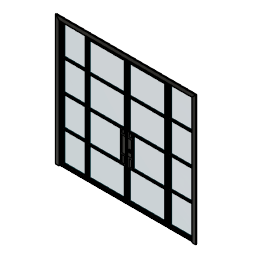
WineDoorModel (Autodesk Fusion 360 design; units mm, degrees)
Autodesk Fusion 360 part; units mm, degrees
note: some values were not read from the file. Set by a fixed rule: which sketch regions a step uses.
(part 1 of 2)
sketch "SubFloor+Framing" plane through (0, 0, 0) normal (0, 1, 0) x (1, 0, 0)
  line L0 (-1333.5, 0) -> (1333.5, 0)
  line L1 (1333.5, 0) -> (1333.5, -2514.6)
  line L2 (-1333.5, 0) -> (-1333.5, -2514.6)
  line L3 (-1333.5, -2514.6) -> (1333.5, -2514.6)
  dimension "d3" = 2667
  dimension "d4" = 2514.6
  dimension "d5" = 2514.6
  constraint horizontal L0
  constraint midpoint origin L0
  constraint perpendicular L0 L1
  constraint perpendicular L0 L2
  measures "d3" distance of L0.start L0.end
  measures "d4" distance of L0.end L1.end
  measures "d5" distance of L0.start L2.end
sketch "FinalOpening" plane through (0, 0, 0) normal (0, 1, 0) x (1, 0, 0)
  line L0 (-1333.5, 0) -> (-1333.5, -2514.6)
  line L1 (-1333.5, -2514.6) -> (1333.5, -2514.6)
  line L2 (1333.5, 0) -> (1333.5, -2514.6)
  line L3 (-1319.2125, 0) -> (-1319.2125, -2500.3125)
  line L4 (-1319.2125, -2500.3125) -> (1319.2125, -2500.3125)
  line L5 (1319.2125, 0) -> (1319.2125, -2500.3125)
  line L6 (-1333.5, 0) -> (1333.5, 0)
  line L7 (-1333.5, -19.05) -> (1333.5, -19.05)
  dimension "d9" = 19.05
sketch "Framing" plane through (0, 0, 0) normal (0, 1, 0) x (1, 0, 0)
  line L0 (-1319.2125, -2500.3125) -> (1319.2125, -2500.3125)
  line L1 (-1319.2125, 0) -> (-1319.2125, -2500.3125)
  line L2 (1319.2125, 0) -> (1319.2125, -2500.3125)
  line L3 (1293.8125, 0) -> (1293.8125, -2474.9125)
  line L4 (-1293.8125, -2474.9125) -> (1293.8125, -2474.9125)
  line L5 (-1293.8125, 0) -> (-1293.8125, -2474.9125)
  line L6 (-1370.0125, 0) -> (-1370.0125, -2551.1125)
  line L7 (-1370.0125, -2551.1125) -> (1370.0125, -2551.1125)
  line L8 (1370.0125, 0) -> (1370.0125, -2551.1125)
  line L9 (-1370.0125, 0) -> (-1293.8125, 0)
  line L10 (1293.8125, 0) -> (1370.0125, 0)
  line L11 (1293.8125, -2474.9125) -> (1370.0125, -2551.1125)
  line L12 (-1370.0125, -2551.1125) -> (-1293.8125, -2474.9125)
  line L13 (1293.8125, -19.05) -> (1370.0125, -19.05)
  line L14 (-1333.5, -19.05) -> (1333.5, -19.05)
  line L15 (-1293.8125, -19.05) -> (-1370.0125, -19.05)
  dimension "d11" = 25.4
  dimension "d12" = 50.8
  constraint perpendicular L6 L9
  constraint perpendicular L8 L10
  constraint coincident L3 L13.start
  constraint coincident L8 L13.end
  constraint perpendicular L8 L13
  constraint collinear L13 L14
  constraint coincident L5 L15.start
  constraint coincident L14 L15.start
  constraint coincident L6 L15.end
  constraint perpendicular L6 L15
sketch "1/2 Bar" plane through (0, 0, 0) normal (0, 1, 0) x (1, 0, 0)
  line L0 (-1293.8125, 0) -> (-1293.8125, -2474.9125)
  line L1 (-1293.8125, -2474.9125) -> (1293.8125, -2474.9125)
  line L2 (1293.8125, 0) -> (1293.8125, -2474.9125)
  line L3 (-1333.5, -19.05) -> (1333.5, -19.05)
  line L4 (-1281.1125, 0) -> (-1281.1125, -2462.2125)
  line L5 (-1281.1125, -2462.2125) -> (1281.1125, -2462.2125)
  line L6 (1281.1125, 0) -> (1281.1125, -2462.2125)
  line L7 (-1333.5, -31.75) -> (1333.5, -31.75)
  line L8 (-1319.2125, -2500.3125) -> (1319.2125, -2500.3125)
  line L9 (-1281.1125, -31.75) -> (-1281.1125, -2462.2125)
  line L10 (0, -2462.2125) -> (0, -31.75)
  line L11 (-787.4, -2462.2125) -> (-787.4, -31.75)
  line L12 (-800.1, -2462.2125) -> (-800.1, -31.75)
  line L13 (787.4, -2462.2125) -> (787.4, -31.75)
  line L14 (800.1, -2462.2125) -> (800.1, -31.75)
  dimension "d13" = -12.7
  dimension "d14" = 12.7
  dimension "d50" = 787.4
  dimension "d51" = 12.7
  dimension "d52" = 787.4
  dimension "d53" = 12.7
  constraint coincident L7 L9.start
  constraint coincident L4 L9.start
  constraint midpoint L5 L10.start
  constraint midpoint L7 L10.end
  constraint perpendicular L7 L10
  constraint coincident L5 L11.start
  constraint coincident L7 L11.end
  constraint perpendicular L7 L11
  constraint coincident L5 L12.start
  constraint coincident L7 L12.end
  constraint perpendicular L7 L12
  constraint coincident L5 L13.start
  constraint coincident L7 L13.end
  constraint perpendicular L7 L13
  constraint coincident L5 L14.start
  constraint coincident L7 L14.end
  constraint perpendicular L7 L14
  measures "d50" distance of L10 L11
  measures "d51" distance of L11 L12
  measures "d52" distance of L10 L13
  measures "d53" distance of L13 L14
sketch "SideLights" plane through (0, 0, 0) normal (0, 1, 0) x (1, 0, 0)
  line L0 (-1281.1125, -31.75) -> (-800.1, -31.75)
  line L1 (-800.1, -31.75) -> (-800.1, -2462.2125)
  line L2 (-800.1, -2462.2125) -> (-1281.1125, -2462.2125)
  line L3 (-1281.1125, -2462.2125) -> (-1281.1125, -31.75)
  line L4 (-1249.3625, -63.5) -> (-831.85, -63.5)
  line L5 (-831.85, -2430.4625) -> (-1249.3625, -2430.4625)
  line L6 (-1249.3625, -2430.4625) -> (-1249.3625, -1862.5344)
  line L7 (-1249.3625, -1231.1063) -> (-831.85, -1231.1063)
  line L8 (-1249.3625, -1262.8563) -> (-831.85, -1262.8563)
  line L9 (-1249.3625, -1830.7844) -> (-831.85, -1830.7844)
  line L10 (-1249.3625, -1862.5344) -> (-831.85, -1862.5344)
  line L11 (-1249.3625, -631.4281) -> (-1249.3625, -63.5)
  line L12 (-1249.3625, -1231.1063) -> (-1249.3625, -663.1781)
  line L13 (-1249.3625, -1830.7844) -> (-1249.3625, -1262.8563)
  line L14 (-831.85, -63.5) -> (-831.85, -631.4281)
  line L15 (-831.85, -663.1781) -> (-831.85, -1231.1063)
  line L16 (-831.85, -1262.8563) -> (-831.85, -1830.7844)
  line L17 (-831.85, -1862.5344) -> (-831.85, -2430.4625)
  line L18 (-1249.3625, -663.1781) -> (-831.85, -663.1781)
  line L19 (-1249.3625, -631.4281) -> (-831.85, -631.4281)
  line L20 (0, -2462.2125) -> (0, -31.75)
  line L21 (1249.3625, -1862.5344) -> (831.85, -1862.5344)
  line L22 (831.85, -1862.5344) -> (831.85, -2430.4625)
  line L23 (1249.3625, -2430.4625) -> (1249.3625, -1862.5344)
  line L24 (831.85, -2430.4625) -> (1249.3625, -2430.4625)
  line L25 (800.1, -31.75) -> (800.1, -2462.2125)
  line L26 (800.1, -2462.2125) -> (1281.1125, -2462.2125)
  line L27 (1249.3625, -1830.7844) -> (831.85, -1830.7844)
  line L28 (1281.1125, -31.75) -> (800.1, -31.75)
  line L29 (1249.3625, -663.1781) -> (831.85, -663.1781)
  line L30 (1249.3625, -1231.1062) -> (831.85, -1231.1062)
  line L31 (1249.3625, -1830.7844) -> (1249.3625, -1262.8562)
  line L32 (831.85, -1262.8562) -> (831.85, -1830.7844)
  line L33 (1249.3625, -631.4281) -> (831.85, -631.4281)
  line L34 (1249.3625, -63.5) -> (831.85, -63.5)
  line L35 (1281.1125, -2462.2125) -> (1281.1125, -31.75)
  line L36 (1249.3625, -631.4281) -> (1249.3625, -63.5)
  line L37 (831.85, -63.5) -> (831.85, -631.4281)
  line L38 (1249.3625, -1262.8562) -> (831.85, -1262.8562)
  line L39 (831.85, -663.1781) -> (831.85, -1231.1062)
  line L40 (1249.3625, -1231.1062) -> (1249.3625, -663.1781)
  line L41 (-1040.6062, -2430.4625) -> (-1040.6062, -2462.2125)
  point P0 (-1281.1125, -31.75)
  point P1 (-800.1, -31.75)
  point P2 (-800.1, -2462.2125)
  point P3 (-1281.1125, -2462.2125)
  point P4 (800.1, -2462.2125)
  point P5 (800.1, -31.75)
  point P6 (1281.1125, -2462.2125)
  point P7 (1281.1125, -31.75)
  dimension "d56" = 31.75
  dimension "d57" = 31.75
  dimension "d58" = 31.75
  dimension "d124" = 31.75
  dimension "d129" = 567.9281
  dimension "d130" = 567.9281
  dimension "d131" = 567.9281
  dimension "d132" = 567.9281
  constraint coincident P0 L0.start
  constraint coincident P1 L0.end
  constraint coincident P2 L1.end
  constraint coincident P3 L2.end
  constraint coincident L15.start L14
  constraint coincident L7.end L14
  constraint perpendicular L7 L14
  constraint coincident L8.end L14
  constraint perpendicular L8 L14
  constraint coincident L9.end L14
  constraint perpendicular L9 L14
  constraint coincident L10.end L14
  constraint perpendicular L10 L14
  constraint coincident L12.end L11
  constraint coincident L8.start L12
  constraint coincident L6.end L13
  constraint collinear L14 L15
  constraint collinear L15 L16
  constraint collinear L16 L17
  constraint collinear L6 L13
  constraint perpendicular L15 L18
  constraint perpendicular L14 L19
  constraint collinear L11 L12
  constraint symmetric P0 L20 P7
  constraint symmetric P1 L20 P5
  constraint symmetric P2 L20 P4
  constraint symmetric P3 L20 P6
  constraint symmetric L4.start L20 L34.start
  constraint symmetric L4.end L20 L34.end
  constraint symmetric L5.start L20 L22.end
  constraint symmetric L5.end L20 L23.start
  constraint symmetric L11.start L20 L33.start
  constraint symmetric L14.end L20 L33.end
  constraint symmetric L12.end L20 L29.start
  constraint symmetric L15.start L20 L29.end
  constraint symmetric L7.start L20 L30.start
  constraint symmetric L7.end L20 L30.end
  constraint symmetric L8.start L20 L31.end
  constraint symmetric L8.end L20 L32.start
  constraint symmetric L9.start L20 L27.start
  constraint symmetric L9.end L20 L27.end
  constraint symmetric L6.end L20 L21.start
  constraint symmetric L10.end L20 L21.end
  constraint midpoint L5 L41.start
  constraint midpoint L2 L41.end
  constraint perpendicular L4 L11
  measures "d56" distance of L7 L8
  measures "d57" distance of L9 L10
  measures "d58" distance of L18 L19
  measures "d124" distance of L41.start L41.end
  measures "d129" distance of L5 L10
  measures "d130" distance of L4.start L11.start
  measures "d131" distance of L12.end L7.start
  measures "d132" distance of L8.start L9.start
sketch "Doors" plane through (0, 0, 0) normal (0, 1, 0) x (1, 0, 0)
  line L0 (-787.4, -31.75) -> (787.4, -31.75)
  line L1 (787.4, -31.75) -> (787.4, -2462.2125)
  line L2 (787.4, -2462.2125) -> (-787.4, -2462.2125)
  line L3 (-787.4, -2462.2125) -> (-787.4, -31.75)
  line L4 (-787.4, -2462.2125) -> (-787.4, -31.75)
  line L5 (782.6375, -41.275) -> (782.6375, -2457.45)
  line L6 (782.6375, -2457.45) -> (-782.6375, -2457.45)
  line L7 (-782.6375, -2457.45) -> (-782.6375, -41.275)
  line L8 (-3.175, -41.275) -> (3.175, -41.275)
  line L9 (0, -2457.45) -> (0, -41.275)
  line L10 (3.175, -2457.45) -> (3.175, -41.275)
  line L11 (-3.175, -2457.45) -> (-3.175, -41.275)
  line L12 (3.175, -41.275) -> (782.6375, -41.275)
  line L13 (-782.6375, -41.275) -> (-3.175, -41.275)
  line L14 (-15.875, -2444.75) -> (-769.9375, -2444.75)
  line L15 (-769.9375, -2444.75) -> (-769.9375, -53.975)
  line L16 (-769.9375, -53.975) -> (-15.875, -53.975)
  line L17 (-15.875, -2444.75) -> (-15.875, -53.975)
  line L18 (-738.1875, -85.725) -> (-47.625, -85.725)
  line L19 (-47.625, -2413) -> (-738.1875, -2413)
  line L20 (-738.1875, -631.4281) -> (-47.625, -631.4281)
  line L21 (-738.1875, -1262.8563) -> (-47.625, -1262.8562)
  line L22 (-738.1875, -1830.7844) -> (-47.625, -1830.7844)
  line L23 (-738.1875, -1862.5344) -> (-47.625, -1862.5344)
  line L24 (-1249.3625, -631.4281) -> (-831.85, -631.4281)
  line L25 (-1249.3625, -663.1781) -> (-831.85, -663.1781)
  line L26 (-1249.3625, -1231.1063) -> (-831.85, -1231.1063)
  line L27 (-1249.3625, -1262.8563) -> (-831.85, -1262.8563)
  line L28 (-1249.3625, -1830.7844) -> (-831.85, -1830.7844)
  line L29 (-1249.3625, -1862.5344) -> (-831.85, -1862.5344)
  line L30 (-738.1875, -631.4281) -> (-738.1875, -85.725)
  line L31 (-47.625, -631.4281) -> (-47.625, -85.725)
  line L32 (-738.1875, -1231.1063) -> (-738.1875, -663.1781)
  line L33 (-47.625, -2413) -> (-47.625, -1862.5344)
  line L34 (-47.625, -1830.7844) -> (-47.625, -1262.8562)
  line L35 (-738.1875, -2413) -> (-738.1875, -1862.5344)
  line L36 (-738.1875, -1830.7844) -> (-738.1875, -1262.8563)
  line L37 (15.875, -2444.75) -> (15.875, -53.975)
  line L38 (738.1875, -85.725) -> (47.625, -85.725)
  line L39 (47.625, -631.4281) -> (47.625, -85.725)
  line L40 (769.9375, -53.975) -> (15.875, -53.975)
  line L41 (738.1875, -1262.8563) -> (47.625, -1262.8562)
  line L42 (738.1875, -1231.1063) -> (738.1875, -663.1781)
  line L43 (738.1875, -1830.7844) -> (738.1875, -1262.8563)
  line L44 (47.625, -1830.7844) -> (47.625, -1262.8562)
  line L45 (738.1875, -631.4281) -> (47.625, -631.4281)
  line L46 (738.1875, -631.4281) -> (738.1875, -85.725)
  line L47 (769.9375, -2444.75) -> (769.9375, -53.975)
  line L48 (15.875, -2444.75) -> (769.9375, -2444.75)
  line L49 (738.1875, -2413) -> (738.1875, -1862.5344)
  line L50 (47.625, -2413) -> (738.1875, -2413)
  line L51 (47.625, -2413) -> (47.625, -1862.5344)
  line L52 (738.1875, -1830.7844) -> (47.625, -1830.7844)
  line L53 (738.1875, -1862.5344) -> (47.625, -1862.5344)
  line L54 (125.4125, -1231.1062) -> (125.4125, -663.1781)
  line L55 (47.625, -1167.6063) -> (93.6625, -1167.6063)
  line L56 (93.6625, -1167.6063) -> (93.6625, -1231.1062)
  line L57 (15.875, -1135.8563) -> (93.6625, -1135.8563)
  line L58 (47.625, -1231.1062) -> (47.625, -1167.6063)
  line L59 (47.625, -663.1781) -> (47.625, -799.3063)
  line L60 (15.875, -831.0563) -> (93.6625, -831.0563)
  line L61 (47.625, -799.3063) -> (93.6625, -799.3063)
  line L62 (93.6625, -1135.8563) -> (93.6625, -831.0563)
  line L63 (93.6625, -799.3063) -> (93.6625, -663.1781)
  line L64 (738.1875, -663.1781) -> (125.4125, -663.1781)
  line L65 (93.6625, -663.1781) -> (47.625, -663.1781)
  line L66 (738.1875, -1231.1063) -> (125.4125, -1231.1062)
  line L67 (93.6625, -1231.1062) -> (47.625, -1231.1062)
  line L68 (-47.625, -663.1781) -> (-47.625, -799.3063)
  line L69 (-93.6625, -663.1781) -> (-47.625, -663.1781)
  line L70 (-93.6625, -799.3063) -> (-93.6625, -663.1781)
  line L71 (-47.625, -799.3063) -> (-93.6625, -799.3063)
  line L72 (-93.6625, -1167.6063) -> (-93.6625, -1231.1062)
  line L73 (-93.6625, -1231.1062) -> (-47.625, -1231.1062)
  line L74 (-47.625, -1167.6063) -> (-93.6625, -1167.6063)
  line L75 (-47.625, -1231.1062) -> (-47.625, -1167.6063)
  line L76 (-93.6625, -1135.8563) -> (-93.6625, -831.0563)
  line L77 (-15.875, -1135.8563) -> (-93.6625, -1135.8563)
  line L78 (-15.875, -831.0563) -> (-93.6625, -831.0563)
  line L79 (-125.4125, -1231.1062) -> (-125.4125, -663.1781)
  line L80 (-47.625, -799.3063) -> (-47.625, -663.1781)
  line L81 (-738.1875, -663.1781) -> (-125.4125, -663.1781)
  line L82 (-93.6625, -663.1781) -> (-47.625, -663.1781)
  line L83 (-47.625, -1231.1062) -> (-47.625, -1167.6063)
  line L84 (-738.1875, -1231.1063) -> (-125.4125, -1231.1062)
  line L85 (-93.6625, -1231.1062) -> (-47.625, -1231.1062)
  point P0 (-787.4, -31.75)
  point P1 (787.4, -31.75)
  point P2 (787.4, -2462.2125)
  point P3 (-787.4, -2462.2125)
  dimension "d100" = 3.175
  dimension "d111" = 109.5375
  dimension "d113" = 31.75
  dimension "d114" = 63.5
  dimension "d115" = 31.75
  dimension "d116" = 31.75
  dimension "d117" = 304.8
  constraint coincident P0 L0.start
  constraint coincident P1 L0.end
  constraint coincident P2 L1.end
  constraint coincident P3 L2.end
  constraint midpoint L6 L9.start
  constraint coincident L6 L10.start
  constraint coincident L6 L11.start
  constraint coincident L8 L9.end
  constraint coincident L8.start L12
  constraint coincident L9.end L13
  constraint vertical L9
  constraint coincident L20.start L35
  constraint coincident L20.end L33
  constraint perpendicular L20 L33
  constraint perpendicular L33 L81
  constraint coincident L32.start L35
  constraint coincident L73.end L33
  constraint perpendicular L33 L84
  constraint perpendicular L21 L33
  constraint coincident L22.start L35
  constraint coincident L22.end L33
  constraint perpendicular L22 L33
  constraint perpendicular L23 L33
  constraint collinear L20 L24
  constraint collinear L25 L81
  constraint collinear L26 L84
  constraint collinear L21 L27
  constraint collinear L22 L28
  constraint collinear L23 L29
  constraint collinear L30 L35
  constraint collinear L31 L33
  constraint collinear L32 L35
  constraint collinear L33 L83
  constraint collinear L33 L34
  constraint collinear L35 L36
  constraint symmetric L9 L14.start L37.start
  constraint symmetric L9 L14.end L47.start
  constraint symmetric L9 L15.end L40.start
  constraint symmetric L9 L16.end L37.end
  constraint symmetric L9 L18.start L38.start
  constraint symmetric L9 L18.end L38.end
  constraint symmetric L9 L19.start L50.start
  constraint symmetric L9 L19.end L49.start
  constraint symmetric L9 L20.start L45.start
  constraint symmetric L9 L20.end L39.start
  constraint symmetric L9 L32.end L42.end
  constraint symmetric L9 L68.start L59.start
  constraint symmetric L9 L32.start L42.start
  constraint symmetric L9 L73.end L58.start
  constraint symmetric L9 L21.start L41.start
  constraint symmetric L9 L21.end L41.end
  constraint symmetric L9 L22.start L43.start
  constraint symmetric L9 L22.end L44.start
  constraint symmetric L9 L23.start L49.end
  constraint symmetric L9 L23.end L51.end
  constraint perpendicular L54 L64
  constraint perpendicular L54 L55
  constraint coincident L56.end L66
  constraint perpendicular L56 L66
  constraint coincident L37 L57.start
  constraint perpendicular L54 L57
  constraint perpendicular L55 L58
  constraint perpendicular L57 L62
  constraint collinear L56 L62
  constraint perpendicular L59 L64
  constraint coincident L63.end L64
  constraint coincident L37 L60.start
  constraint perpendicular L54 L60
  constraint coincident L61.end L62
  constraint perpendicular L61 L62
  constraint collinear L62 L63
  constraint collinear L64 L65
  constraint collinear L66 L67
  constraint symmetric L9 L59.start L68.start
  constraint symmetric L9 L58.start L73.end
  constraint symmetric L9 L55.end L72.start
  constraint symmetric L9 L56.end L72.end
  constraint symmetric L9 L57.start L77.start
  constraint symmetric L9 L55.start L74.start
  constraint symmetric L9 L57.end L76.start
  constraint symmetric L9 L63.end L69.start
  constraint symmetric L9 L60.start L78.start
  constraint symmetric L9 L59.end L68.end
  constraint symmetric L9 L61.end L70.start
  constraint symmetric L9 L60.end L76.end
  constraint symmetric L9 L54.start L79.start
  constraint symmetric L9 L54.end L79.end
  constraint collinear L80 L83
  constraint collinear L81 L82
  constraint collinear L84 L85
  measures "d100" distance of L9 L10
  measures "d111" distance of L37 L54
  measures "d113" distance of L54 L56
  measures "d114" distance of L55 L66
  measures "d115" distance of L55 L57
  measures "d116" distance of L60 L61
  measures "d117" distance of L57 L60
extrude "Extrude1" add sketch "Framing" against normal blind 19.05 contours L1 L6 L12 L14 L15 | L1 L5 L12 L14 L15 | L2 L3 L11 L13 L14 | L2 L8 L11 L13 L14 makes body 1 at (-1344.6125, 0, 1681.6917) makes body 2 at (1344.6125, 0, 1681.6917)
extrude "Extrude2" add sketch "Framing" against normal blind 19.05 separate body contours L0 L4 L11 L12 | L0 L7 L11 L12 makes body 3
extrude "Extrude3" add sketch "1/2 Bar" along normal blind 76.2 separate body contours L0 L3 L4 L7 | L0 L1 L2 L4 L5 L6 L7 L9 | L3 L4 L6 L7 | L2 L3 L6 L7 makes body 4
extrude "Extrude4" add sketch "1/2 Bar" along normal blind 76.2 separate body contours L5 L7 L11 L12 | L5 L7 L13 L14 makes body 5 at (-787.4, 50.8, 1652.0583) makes body 6 at (800.1, 50.8, 1652.0583)
extrude "Extrude6" add sketch "SideLights" along normal blind 4.7625 from surface at 26.9875 separate body makes body 7 at (1270.5292, 26.9875, 1041.7969) makes body 8 at (-1270.5292, 26.9875, 1041.7969)
extrude "Extrude7" add sketch "Doors" along normal blind 38.1 separate body contours L5 L6 L10 L12 | L6 L7 L11 L13 makes body 9 at (-3.175, 12.7, 1652.0583) makes body 10 at (782.6375, 12.7, 846.6667)
extrude "Extrude8" add sketch "Doors" along normal blind 4.7625 from surface at 7.9375 separate body contours L14 L15 L16 L17 L76 L77 L78 | L37 L40 L47 L48 L57 L60 L62 makes body 11 at (759.3542, 7.9375, 1453.7531) makes body 12 at (-759.3542, 7.9375, 1453.7531)
sketch "Door Handle Plates" plane through (0, 7.9375, 0) normal (0, -1, 0) x (1, 0, 0)
  line L0 (15.875, 2444.75) -> (15.875, 1135.8563)
  line L1 (15.875, 1254.9187) -> (117.475, 1254.9187)
  line L2 (15.875, 831.0563) -> (15.875, 53.975)
  line L3 (15.875, 639.3656) -> (117.475, 639.3656)
  line L4 (117.475, 1254.9187) -> (117.475, 639.3656)
  line L5 (47.625, 1262.8562) -> (738.1875, 1262.8563)
  line L6 (738.1875, 631.4281) -> (47.625, 631.4281)
  line L7 (15.875, 1254.9187) -> (15.875, 639.3656)
  line L8 (0, 2457.45) -> (0, 41.275)
  line L9 (-15.875, 639.3656) -> (-117.475, 639.3656)
  line L10 (-15.875, 1254.9187) -> (-15.875, 639.3656)
  line L11 (-15.875, 1254.9187) -> (-117.475, 1254.9187)
  line L12 (-117.475, 1254.9187) -> (-117.475, 639.3656)
  point P0 (-15.875, 1135.8563)
  point P1 (-47.625, 1262.8562)
  point P2 (-47.625, 631.4281)
  point P3 (-15.875, 831.0563)
  dimension "d118" = 101.6
  dimension "d119" = 101.6
  dimension "d120" = 7.9375
  dimension "d121" = 7.9375
  constraint coincident L0 L1.start
  constraint perpendicular L0 L1
  constraint horizontal L3
  constraint coincident L2 L3.start
  constraint perpendicular L3 L4
  constraint symmetric L0.end L8 P0
  constraint symmetric L1.start L8 L10.start
  constraint symmetric L1.end L8 L11.end
  constraint symmetric L2.start L8 P3
  constraint symmetric L3.start L8 L9.start
  constraint symmetric L3.end L8 L9.end
  constraint symmetric L5.start L8 P1
  constraint symmetric L6.end L8 P2
  measures "d118" distance of L3.start L3.end
  measures "d119" distance of L1.start L1.end
  measures "d120" distance of L1 L5
  measures "d121" distance of L3 L6
extrude "Extrude9" add sketch "Door Handle Plates" along normal blind 4.7625 separate body makes body 13 at (49.7417, 7.9375, 1049.7344) makes body 14 at (-49.7417, 7.9375, 844.55)
copy_body "CopyPasteBodies1" bodies 12 8 11 7 makes body 15 makes body 16 makes body 17 makes body 18
move_body "Move1" bodies 15 16 17 18 to x (1, 0, 0) y (0, 1, 0) z (0, 0, 1) at (0, 17.4625, 0)
sketch "Sidelight Glass" plane through (0, 31.75, 0) normal (0, 1, 0) x (-1, 0, 0)
  line L0 (-831.85, 63.5) -> (-1249.3625, 63.5)
  line L1 (-831.85, 631.4281) -> (-831.85, 63.5)
  line L2 (-1249.3625, 631.4281) -> (-831.85, 631.4281)
  line L3 (-1249.3625, 63.5) -> (-1249.3625, 631.4281)
  line L4 (-831.85, 663.1781) -> (-1249.3625, 663.1781)
  line L5 (-831.85, 1231.1062) -> (-831.85, 663.1781)
  line L6 (-1249.3625, 1231.1062) -> (-831.85, 1231.1062)
  line L7 (-1249.3625, 663.1781) -> (-1249.3625, 1231.1062)
  line L8 (-831.85, 1262.8562) -> (-1249.3625, 1262.8562)
  line L9 (-831.85, 1830.7844) -> (-831.85, 1262.8562)
  line L10 (-1249.3625, 1830.7844) -> (-831.85, 1830.7844)
  line L11 (-1249.3625, 1262.8562) -> (-1249.3625, 1830.7844)
  line L12 (-1249.3625, 1862.5344) -> (-1249.3625, 2430.4625)
  line L13 (-831.85, 1862.5344) -> (-1249.3625, 1862.5344)
  line L14 (-831.85, 2430.4625) -> (-831.85, 1862.5344)
  line L15 (-1249.3625, 2430.4625) -> (-831.85, 2430.4625)
  line L16 (-800.1, 2462.2125) -> (-1281.1125, 2462.2125)
  line L17 (-800.1, 31.75) -> (-800.1, 2462.2125)
  line L18 (-1281.1125, 31.75) -> (-800.1, 31.75)
  line L19 (-1281.1125, 2462.2125) -> (-1281.1125, 31.75)
  line L20 (-815.975, 2438.4) -> (-815.975, 1854.5969)
  line L21 (-1265.2375, 2438.4) -> (-815.975, 2438.4)
  line L22 (-1265.2375, 1854.5969) -> (-1265.2375, 2438.4)
  line L23 (-815.975, 1854.5969) -> (-1265.2375, 1854.5969)
  line L24 (-815.975, 1838.7219) -> (-815.975, 1254.9187)
  line L25 (-1265.2375, 1254.9187) -> (-1265.2375, 1838.7219)
  line L26 (-815.975, 1239.0437) -> (-815.975, 655.2406)
  line L27 (-1265.2375, 655.2406) -> (-1265.2375, 1239.0437)
  line L28 (-1265.2375, 55.5625) -> (-1265.2375, 639.3656)
  line L29 (-815.975, 639.3656) -> (-815.975, 55.5625)
  line L30 (-1265.2375, 639.3656) -> (-815.975, 639.3656)
  line L31 (-815.975, 55.5625) -> (-1265.2375, 55.5625)
  line L32 (-815.975, 655.2406) -> (-1265.2375, 655.2406)
  line L33 (-1265.2375, 1239.0437) -> (-815.975, 1239.0437)
  line L34 (-815.975, 1254.9187) -> (-1265.2375, 1254.9187)
  line L35 (-1265.2375, 1838.7219) -> (-815.975, 1838.7219)
  line L36 (0, 2457.45) -> (0, 41.275)
  line L37 (1265.2375, 655.2406) -> (1265.2375, 1239.0437)
  line L38 (815.975, 1239.0437) -> (815.975, 655.2406)
  line L39 (1281.1125, 31.75) -> (800.1, 31.75)
  line L40 (1265.2375, 1239.0437) -> (815.975, 1239.0437)
  line L41 (1265.2375, 1254.9187) -> (1265.2375, 1838.7219)
  line L42 (831.85, 1231.1063) -> (831.85, 663.1781)
  line L43 (1249.3625, 1262.8562) -> (1249.3625, 1830.7844)
  line L44 (1265.2375, 55.5625) -> (1265.2375, 639.3656)
  line L45 (1281.1125, 2462.2125) -> (1281.1125, 31.75)
  line L46 (800.1, 31.75) -> (800.1, 2462.2125)
  line L47 (831.85, 1262.8563) -> (1249.3625, 1262.8562)
  line L48 (815.975, 655.2406) -> (1265.2375, 655.2406)
  line L49 (1249.3625, 63.5) -> (1249.3625, 631.4281)
  line L50 (831.85, 631.4281) -> (831.85, 63.5)
  line L51 (1249.3625, 1231.1062) -> (831.85, 1231.1063)
  line L52 (815.975, 1254.9188) -> (1265.2375, 1254.9187)
  line L53 (815.975, 55.5625) -> (1265.2375, 55.5625)
  line L54 (800.1, 2462.2125) -> (1281.1125, 2462.2125)
  line L55 (815.975, 1854.5969) -> (1265.2375, 1854.5969)
  line L56 (815.975, 1838.7219) -> (815.975, 1254.9188)
  line L57 (815.975, 639.3656) -> (815.975, 55.5625)
  line L58 (1249.3625, 631.4281) -> (831.85, 631.4281)
  line L59 (1265.2375, 1854.5969) -> (1265.2375, 2438.4)
  line L60 (831.85, 1830.7844) -> (831.85, 1262.8563)
  line L61 (815.975, 2438.4) -> (815.975, 1854.5969)
  line L62 (1265.2375, 1838.7219) -> (815.975, 1838.7219)
  line L63 (1249.3625, 1862.5344) -> (1249.3625, 2430.4625)
  line L64 (1249.3625, 663.1781) -> (1249.3625, 1231.1062)
  line L65 (1249.3625, 1830.7844) -> (831.85, 1830.7844)
  line L66 (1249.3625, 2430.4625) -> (831.85, 2430.4625)
  line L67 (831.85, 1862.5344) -> (1249.3625, 1862.5344)
  line L68 (831.85, 2430.4625) -> (831.85, 1862.5344)
  line L69 (831.85, 663.1781) -> (1249.3625, 663.1781)
  line L70 (1265.2375, 2438.4) -> (815.975, 2438.4)
  line L71 (1265.2375, 639.3656) -> (815.975, 639.3656)
  line L72 (831.85, 63.5) -> (1249.3625, 63.5)
  line L73 (-800.1, 31.75) -> (-800.1, 2462.2125)
  dimension "d183" = 15.875
  dimension "d184" = 15.875
  dimension "d185" = 15.875
  dimension "d186" = 15.875
  dimension "d187" = 15.875
  dimension "d188" = 15.875
  dimension "d189" = 15.875
  dimension "d190" = 15.875
  dimension "d200" = 23.8125
  dimension "d201" = 23.8125
  dimension "d203" = 15.875
  dimension "d204" = 7.9375
  dimension "d205" = 7.9375
  dimension "d206" = 7.9375
  dimension "d207" = 7.9375
  dimension "d208" = 7.9375
  constraint symmetric L0.start L36 L50.end
  constraint symmetric L0.end L36 L49.start
  constraint symmetric L1.start L36 L50.start
  constraint symmetric L2.start L36 L49.end
  constraint symmetric L4.start L36 L42.end
  constraint symmetric L4.end L36 L64.start
  constraint symmetric L5.start L36 L42.start
  constraint symmetric L6.start L36 L51.start
  constraint symmetric L8.start L36 L47.start
  constraint symmetric L8.end L36 L43.start
  constraint symmetric L9.start L36 L60.start
  constraint symmetric L10.start L36 L43.end
  constraint symmetric L12.start L36 L63.start
  constraint symmetric L12.end L36 L63.end
  constraint symmetric L13.start L36 L67.start
  constraint symmetric L14.start L36 L66.end
  constraint symmetric L16.start L36 L46.end
  constraint symmetric L16.end L36 L45.start
  constraint symmetric L17.start L36 L39.end
  constraint symmetric L18.start L36 L39.start
  constraint symmetric L20.start L36 L61.start
  constraint symmetric L21.start L36 L59.end
  constraint symmetric L22.start L36 L55.end
  constraint symmetric L20.end L36 L55.start
  constraint symmetric L24.start L36 L56.start
  constraint symmetric L25.end L36 L41.end
  constraint symmetric L25.start L36 L41.start
  constraint symmetric L24.end L36 L52.start
  constraint symmetric L26.start L36 L38.start
  constraint symmetric L27.end L36 L37.end
  constraint symmetric L27.start L36 L37.start
  constraint symmetric L26.end L36 L38.end
  constraint symmetric L29.start L36 L57.start
  constraint symmetric L28.end L36 L44.end
  constraint symmetric L28.start L36 L44.start
  constraint symmetric L29.end L36 L53.start
  measures "d183" distance of L19 L22
  measures "d184" distance of L19 L25
  measures "d185" distance of L19 L27
  measures "d186" distance of L19 L28
  measures "d187" distance of L17 L29
  measures "d188" distance of L17 L26
  measures "d189" distance of L24 L73
  measures "d190" distance of L20 L73
  measures "d200" distance of L16 L21
  measures "d201" distance of L18 L31
  measures "d203" distance of L33 L34
  measures "d204" distance of L8 L34
  measures "d205" distance of L2 L30
  measures "d206" distance of L4 L32
  measures "d207" distance of L10 L35
  measures "d208" distance of L13 L23
extrude "Extrude10" add sketch "Sidelight Glass" along normal blind 6.35 separate body contours L0 L1 L2 L3 | L4 L5 L6 L7 | L8 L9 L10 L11 | L12 L13 L14 L15 | L20 L21 L22 L23 | L24 L25 L34 L35 | L26 L27 L32 L33 | L28 L29 L30 L31 | L37 L38 L40 L48 | L41 L52 L56 L62 | L42 L51 L64 L69 | L43 L47 L60 L65 | L44 L53 L57 L71 | L49 L50 L58 L72 | L55 L59 L61 L70 | L63 L66 L67 L68 makes body 19 at (-965.7292, 31.75, 1644.1208) makes body 20 at (965.7292, 31.75, 1044.4427) makes body 21 at (965.7292, 31.75, 1644.1208) makes body 22 at (-965.7292, 31.75, 1044.4427) makes body 23 at (-965.7292, 31.75, 2243.799) makes body 24 at (965.7292, 31.75, 444.7646) makes body 25 at (965.7292, 31.75, 2243.799) makes body 26 at (-965.7292, 31.75, 444.7646)
sketch "DoorGlass" plane through (0, 12.7, 0) normal (0, 1, 0) x (-1, 0, 0)
  line L0 (-47.625, 1167.6063) -> (-93.6625, 1167.6063)
  line L1 (-47.625, 1231.1062) -> (-47.625, 1167.6063)
  line L2 (-93.6625, 1231.1062) -> (-47.625, 1231.1062)
  line L3 (-93.6625, 1167.6063) -> (-93.6625, 1231.1062)
  line L4 (-125.4125, 1231.1062) -> (-125.4125, 663.1781)
  line L5 (-738.1875, 1231.1063) -> (-125.4125, 1231.1062)
  line L6 (-738.1875, 663.1781) -> (-738.1875, 1231.1063)
  line L7 (-125.4125, 663.1781) -> (-738.1875, 663.1781)
  line L8 (-47.625, 799.3063) -> (-47.625, 663.1781)
  line L9 (-93.6625, 799.3063) -> (-47.625, 799.3063)
  line L10 (-93.6625, 663.1781) -> (-93.6625, 799.3063)
  line L11 (-738.1875, 1862.5344) -> (-738.1875, 2413)
  line L12 (-47.625, 1862.5344) -> (-738.1875, 1862.5344)
  line L13 (-47.625, 2413) -> (-47.625, 1862.5344)
  line L14 (-738.1875, 2413) -> (-47.625, 2413)
  line L15 (-47.625, 1830.7844) -> (-47.625, 1262.8562)
  line L16 (-738.1875, 1830.7844) -> (-47.625, 1830.7844)
  line L17 (-738.1875, 1262.8563) -> (-738.1875, 1830.7844)
  line L18 (-47.625, 1262.8562) -> (-738.1875, 1262.8563)
  line L19 (-738.1875, 85.725) -> (-738.1875, 631.4281)
  line L20 (-47.625, 85.725) -> (-738.1875, 85.725)
  line L21 (-47.625, 631.4281) -> (-47.625, 85.725)
  line L22 (-738.1875, 631.4281) -> (-47.625, 631.4281)
  line L23 (-15.875, 2444.75) -> (-15.875, 1135.8563)
  line L24 (-15.875, 1135.8563) -> (-93.6625, 1135.8563)
  line L25 (-93.6625, 1135.8563) -> (-93.6625, 831.0563)
  line L26 (-15.875, 831.0563) -> (-93.6625, 831.0563)
  line L27 (-15.875, 831.0563) -> (-15.875, 53.975)
  line L28 (-769.9375, 53.975) -> (-15.875, 53.975)
  line L29 (-769.9375, 2444.75) -> (-769.9375, 53.975)
  line L30 (-15.875, 2444.75) -> (-769.9375, 2444.75)
  line L31 (125.4125, 1231.1062) -> (738.1875, 1231.1063)
  line L32 (125.4125, 663.1781) -> (125.4125, 1231.1062)
  line L33 (738.1875, 663.1781) -> (125.4125, 663.1781)
  line L34 (738.1875, 1231.1063) -> (738.1875, 663.1781)
  line L35 (47.625, 1167.6063) -> (47.625, 1231.1062)
  line L36 (93.6625, 1167.6063) -> (47.625, 1167.6063)
  line L37 (93.6625, 1231.1062) -> (93.6625, 1167.6063)
  line L38 (47.625, 1231.1062) -> (93.6625, 1231.1062)
  line L39 (93.6625, 799.3063) -> (93.6625, 663.1781)
  line L40 (47.625, 799.3063) -> (93.6625, 799.3063)
  line L41 (47.625, 663.1781) -> (47.625, 799.3063)
  line L42 (738.1875, 1262.8563) -> (47.625, 1262.8562)
  line L43 (738.1875, 1830.7844) -> (738.1875, 1262.8563)
  line L44 (47.625, 1830.7844) -> (738.1875, 1830.7844)
  line L45 (47.625, 1262.8562) -> (47.625, 1830.7844)
  line L46 (738.1875, 1862.5344) -> (47.625, 1862.5344)
  line L47 (738.1875, 2413) -> (738.1875, 1862.5344)
  line L48 (47.625, 2413) -> (738.1875, 2413)
  line L49 (47.625, 1862.5344) -> (47.625, 2413)
  line L50 (47.625, 85.725) -> (47.625, 631.4281)
  line L51 (738.1875, 85.725) -> (47.625, 85.725)
  line L52 (738.1875, 631.4281) -> (738.1875, 85.725)
  line L53 (47.625, 631.4281) -> (738.1875, 631.4281)
  line L54 (15.875, 2444.75) -> (769.9375, 2444.75)
  line L55 (769.9375, 2444.75) -> (769.9375, 53.975)
  line L56 (769.9375, 53.975) -> (15.875, 53.975)
  line L57 (15.875, 831.0563) -> (15.875, 53.975)
  line L58 (15.875, 831.0563) -> (93.6625, 831.0563)
  line L59 (93.6625, 1135.8563) -> (93.6625, 831.0563)
  line L60 (15.875, 1135.8563) -> (93.6625, 1135.8563)
  line L61 (15.875, 2444.75) -> (15.875, 1135.8563)
  line L62 (-31.75, 1838.7219) -> (-31.75, 1254.9187)
  line L63 (-31.75, 2420.9375) -> (-31.75, 1854.5969)
  line L64 (-754.0625, 1854.5969) -> (-754.0625, 2420.9375)
  line L65 (-754.0625, 1254.9188) -> (-754.0625, 1838.7219)
  line L66 (-754.0625, 655.2406) -> (-754.0625, 1239.0438)
  line L67 (-109.5375, 1239.0437) -> (-109.5375, 655.2406)
  line L68 (-754.0625, 77.7875) -> (-754.0625, 639.3656)
  line L69 (-31.75, 639.3656) -> (-31.75, 77.7875)
  line L70 (-31.75, 77.7875) -> (-754.0625, 77.7875)
  line L71 (-754.0625, 639.3656) -> (-31.75, 639.3656)
  line L72 (-109.5375, 655.2406) -> (-754.0625, 655.2406)
  line L73 (-754.0625, 1239.0438) -> (-109.5375, 1239.0437)
  line L74 (-31.75, 1254.9187) -> (-754.0625, 1254.9188)
  line L75 (-754.0625, 1838.7219) -> (-31.75, 1838.7219)
  line L76 (-31.75, 1854.5969) -> (-754.0625, 1854.5969)
  line L77 (-754.0625, 2420.9375) -> (-31.75, 2420.9375)
  line L78 (0, 2457.45) -> (0, 41.275)
  line L79 (738.1875, 631.4281) -> (47.625, 631.4281)
  line L80 (31.75, 2420.9375) -> (31.75, 1854.5969)
  line L81 (47.625, 1262.8562) -> (738.1875, 1262.8563)
  line L82 (754.0625, 2420.9375) -> (31.75, 2420.9375)
  line L83 (754.0625, 639.3656) -> (31.75, 639.3656)
  line L84 (47.625, 799.3063) -> (47.625, 663.1781)
  line L85 (754.0625, 77.7875) -> (754.0625, 639.3656)
  line L86 (93.6625, 799.3063) -> (47.625, 799.3063)
  line L87 (15.875, 831.0563) -> (93.6625, 831.0563)
  line L88 (31.75, 639.3656) -> (31.75, 77.7875)
  line L89 (47.625, 2413) -> (47.625, 1862.5344)
  line L90 (47.625, 631.4281) -> (47.625, 85.725)
  line L91 (47.625, 663.1781) -> (93.6625, 663.1781)
  line L92 (15.875, 2444.75) -> (769.9375, 2444.75)
  line L93 (47.625, 1231.1062) -> (47.625, 1167.6063)
  line L94 (47.625, 1862.5344) -> (738.1875, 1862.5344)
  line L95 (15.875, 831.0563) -> (15.875, 53.975)
  line L96 (738.1875, 2413) -> (47.625, 2413)
  line L97 (769.9375, 53.975) -> (15.875, 53.975)
  line L98 (15.875, 1135.8563) -> (93.6625, 1135.8563)
  line L99 (754.0625, 1854.5969) -> (754.0625, 2420.9375)
  line L100 (738.1875, 1231.1063) -> (125.4125, 1231.1062)
  line L101 (738.1875, 1830.7844) -> (47.625, 1830.7844)
  line L102 (93.6625, 1167.6063) -> (93.6625, 1231.1062)
  line L103 (31.75, 77.7875) -> (754.0625, 77.7875)
  line L104 (738.1875, 1862.5344) -> (738.1875, 2413)
  line L105 (754.0625, 1838.7219) -> (31.75, 1838.7219)
  line L106 (31.75, 1854.5969) -> (754.0625, 1854.5969)
  line L107 (93.6625, 1231.1062) -> (47.625, 1231.1062)
  line L108 (47.625, 85.725) -> (738.1875, 85.725)
  line L109 (738.1875, 85.725) -> (738.1875, 631.4281)
  line L110 (109.5375, 655.2406) -> (754.0625, 655.2406)
  line L111 (769.9375, 2444.75) -> (769.9375, 53.975)
  line L112 (31.75, 1838.7219) -> (31.75, 1254.9187)
  line L113 (31.75, 1254.9187) -> (754.0625, 1254.9188)
  line L114 (754.0625, 1254.9188) -> (754.0625, 1838.7219)
  line L115 (47.625, 1830.7844) -> (47.625, 1262.8562)
  line L116 (754.0625, 655.2406) -> (754.0625, 1239.0438)
  line L117 (125.4125, 663.1781) -> (738.1875, 663.1781)
  line L118 (15.875, 2444.75) -> (15.875, 1135.8563)
  line L119 (47.625, 1167.6063) -> (93.6625, 1167.6063)
  line L120 (93.6625, 1135.8563) -> (93.6625, 831.0563)
  line L121 (754.0625, 1239.0438) -> (109.5375, 1239.0437)
  line L122 (93.6625, 663.1781) -> (93.6625, 799.3063)
  line L123 (109.5375, 1239.0437) -> (109.5375, 655.2406)
  line L124 (738.1875, 1262.8563) -> (738.1875, 1830.7844)
  line L125 (-47.625, 663.1781) -> (-93.6625, 663.1781)
  line L126 (93.6625, 663.1781) -> (47.625, 663.1781)
  dimension "d191" = 15.875
  dimension "d192" = 15.875
  dimension "d193" = 15.875
  dimension "d194" = 15.875
  dimension "d209" = 7.9375
  dimension "d210" = 7.9375
  dimension "d211" = 7.9375
  dimension "d212" = 7.9375
  dimension "d213" = 7.9375
  dimension "d214" = 7.9375
  dimension "d215" = 7.9375
  constraint symmetric L0.start L78 L35.start
  constraint symmetric L0.end L78 L36.start
  constraint symmetric L1.start L78 L35.end
  constraint symmetric L2.start L78 L37.start
  constraint symmetric L4.start L78 L31.start
  constraint symmetric L4.end L78 L32.start
  constraint symmetric L5.start L78 L31.end
  constraint symmetric L6.start L78 L33.start
  constraint symmetric L8.start L78 L40.start
  constraint symmetric L8.end L78 L41.start
  constraint symmetric L9.start L78 L39.start
  constraint symmetric L10.start L78 L39.end
  constraint symmetric L11.start L78 L46.start
  constraint symmetric L11.end L78 L47.start
  constraint symmetric L12.start L78 L46.end
  constraint symmetric L13.start L78 L48.start
  constraint symmetric L15.start L78 L44.start
  constraint symmetric L15.end L78 L42.end
  constraint symmetric L16.start L78 L43.start
  constraint symmetric L17.start L78 L42.start
  constraint symmetric L19.start L78 L51.start
  constraint symmetric L19.end L78 L52.start
  constraint symmetric L20.start L78 L50.start
  constraint symmetric L21.start L78 L50.end
  constraint symmetric L23.start L78 L54.start
  constraint symmetric L23.end L78 L60.start
  constraint symmetric L24.end L78 L59.start
  constraint symmetric L25.end L78 L58.end
  constraint symmetric L26.start L78 L57.start
  constraint symmetric L27.end L78 L56.end
  constraint symmetric L28.start L78 L55.end
  constraint symmetric L29.start L78 L54.end
  constraint symmetric L69.end L78 L88.end
  constraint symmetric L68.start L78 L85.start
  constraint symmetric L68.end L78 L83.start
  constraint symmetric L69.start L78 L83.end
  constraint symmetric L66.start L78 L110.end
  constraint symmetric L67.end L78 L110.start
  constraint symmetric L67.start L78 L121.end
  constraint symmetric L66.end L78 L116.end
  constraint symmetric L65.start L78 L113.end
  constraint symmetric L62.end L78 L112.end
  constraint symmetric L62.start L78 L105.end
  constraint symmetric L65.end L78 L105.start
  constraint symmetric L64.start L78 L99.start
  constraint symmetric L63.end L78 L80.end
  constraint symmetric L63.start L78 L80.start
  constraint symmetric L64.end L78 L82.start
  measures "d191" distance of L29 L68
  measures "d192" distance of L29 L66
  measures "d193" distance of L29 L65
  measures "d194" distance of L29 L64
  measures "d209" distance of L14 L77
  measures "d210" distance of L12 L76
  measures "d211" distance of L16 L75
  measures "d212" distance of L5 L73
  measures "d213" distance of L18 L74
  measures "d214" distance of L7 L72
  measures "d215" distance of L22 L71
extrude "Extrude11" add sketch "DoorGlass" along normal blind 6.35 separate body contours L4 L5 L6 L7 | L11 L12 L13 L14 | L15 L16 L17 L18 | L19 L20 L21 L22 | L31 L32 L33 L34 L100 L117 | L42 L43 L44 L45 L81 L101 L115 L124 | L46 L47 L48 L49 L89 L94 L96 L104 | L50 L51 L52 L53 L79 L90 L108 L109 | L62 L65 L74 L75 | L63 L64 L76 L77 | L66 L67 L72 L73 | L68 L69 L70 L71 | L80 L82 L99 L106 | L83 L85 L88 L103 | L105 L112 L113 L114 | L110 L116 L121 L123 makes body 27 at (-272.5208, 12.7, 1449.5198) makes body 28 at (324.3792, 12.7, 849.8417) makes body 29 at (272.5208, 12.7, 1449.5198) makes body 30 at (-324.3792, 12.7, 849.8417) makes body 31 at (-513.2917, 12.7, 2232.1573) makes body 32 at (513.2917, 12.7, 264.9802) makes body 33 at (513.2917, 12.7, 2232.1573) makes body 34 at (-513.2917, 12.7, 264.9802)
sketch "Sketch14" plane through (0, 0, 0) normal (0, 1, 0) x (1, 0, 0)
  line L0 (117.475, -1254.9187) -> (15.875, -1254.9187)
  line L1 (15.875, -1254.9187) -> (15.875, -639.3656)
  line L2 (15.875, -639.3656) -> (117.475, -639.3656)
  line L3 (117.475, -639.3656) -> (117.475, -1254.9187)
  line L4 (-1293.8125, -19.05) -> (1293.8125, -19.05)
  circle A0 centre (60.325, -933.45) radius 28.575
  dimension "d197" = 57.15
  dimension "d198" = 914.4
  dimension "d199" = 57.15
  measures "d197" diameter of A0
  measures "d198" distance of L4 A0.centre
  measures "d199" distance of L3 A0.centre
extrude "Extrude12" cut sketch "Sketch14" along normal blind 1270 contours A0 bodies 13
copy_body "CopyPasteBodies2" bodies 14 13 makes body 35 makes body 36
move_body "Move2" bodies 35 36 to x (1, 0, 0) y (0, 1, 0) z (0, 0, 1) at (0, 38.1, 0)
move_body "Align1" bodies 36 to x (1, 0, 0) y (0, 1, 0) z (0, 0, 1) at (0, -11.1125, 0)
move_body "Align2" bodies 35 to x (1, 0, 0) y (0, 1, 0) z (0, 0, 1) at (0, -11.1125, 0)
move_body "Move5" bodies 18 17 15 16 36 35 to x (1, 0, 0) y (0, 1, 0) z (0, 0, 1) at (0, -6.35, 0)
sketch "Top Down?" plane through (0, 0, 0) normal (0, 0, 1) x (1, 0, 0)
  line L0 (1293.8125, 0) -> (1293.8125, 76.2)
  line L1 (-1293.8125, 0) -> (-1293.8125, 76.2)
  line L2 (-1293.8125, 0) -> (1293.8125, 0)
  line L3 (1293.8125, 76.2) -> (-1293.8125, 76.2)
  line L4 (1293.8125, 0) -> (1370.0125, 0)
  line L5 (1370.0125, 0) -> (1370.0125, -19.05)
  line L6 (1293.8125, -19.05) -> (1370.0125, -19.05)
  line L7 (-1293.8125, 0) -> (1293.8125, 0)
  line L8 (-1293.8125, -19.05) -> (1293.8125, -19.05)
  line L9 (-1370.0125, 0) -> (-1293.8125, 0)
  line L10 (-1370.0125, -19.05) -> (-1293.8125, -19.05)
  line L11 (-1370.0125, 0) -> (-1370.0125, -19.05)
  line L12 (1293.8125, 0) -> (1293.8125, -19.05)
  line L13 (1370.0125, 0) -> (1370.0125, -19.05)
  line L14 (1293.8125, 0) -> (1370.0125, 0)
  line L15 (1293.8125, -19.05) -> (1370.0125, -19.05)
  line L16 (-1370.0125, 0) -> (-1370.0125, -19.05)
  line L17 (-1293.8125, 0) -> (-1293.8125, -19.05)
  line L18 (-1293.8125, 0) -> (-1370.0125, 0)
  line L19 (-1370.0125, -19.05) -> (-1293.8125, -19.05)
  line L20 (-787.4, 0) -> (-787.4, 76.2)
  line L21 (-787.4, 76.2) -> (-787.4, 0)
  line L22 (-782.6375, 0) -> (-782.6375, 38.1)
  line L23 (-782.6375, 38.1) -> (-782.6375, 0)
  line L24 (787.4, 0) -> (787.4, 76.2)
  line L25 (787.4, 76.2) -> (787.4, 0)
  line L26 (782.6375, 0) -> (782.6375, 38.1)
  line L27 (782.6375, 38.1) -> (782.6375, 0)
  circle A0 centre (785.0187, -7.5719) radius 7.9375
  dimension "d179" = 15.875
  constraint coincident L26.start A0
  constraint coincident L24.start A0
  measures "d179" diameter of A0
sketch "Sketch15" plane through (0, 0, 0) normal (0, -1, 0) x (1, 0, 0)
  line L0 (3.175, 2457.45) -> (-3.175, 2457.45)
  line L1 (-12.7, 2457.45) -> (12.7, 2457.45)
  line L2 (3.175, 41.275) -> (-3.175, 41.275)
  line L3 (-12.7, 41.275) -> (12.7, 41.275)
  line L4 (-12.7, 41.275) -> (-12.7, 2457.45)
  line L5 (12.7, 2457.45) -> (12.7, 41.275)
  point P0 (3.175, 2457.45)
  point P1 (-3.175, 2457.45)
  point P2 (3.175, 41.275)
  point P3 (-3.175, 41.275)
  dimension "d217" = 25.4
  dimension "d218" = 25.4
  constraint coincident P0 L0.start
  constraint coincident P1 L0.end
  constraint horizontal L1
  constraint midpoint L0 L1
  constraint coincident P2 L2.start
  constraint coincident P3 L2.end
  constraint horizontal L3
  constraint midpoint L2 L3
  measures "d217" distance of L1.start L1.end
  measures "d218" distance of L3.start L3.end
extrude "Extrude14" add sketch "Sketch15" along normal blind 4.7625 separate body makes body 37
copy_body "Body->Comp1" bodies 19 removing the originals makes body 38 in component "Component"
copy_body "Body->Comp2" bodies 26 removing the originals makes body 39 in component "Component'"
copy_body "Body->Comp3" bodies 22 removing the originals makes body 40 in component "Component''"
copy_body "Body->Comp4" bodies 21 removing the originals makes body 41 in component "Component'''"
copy_body "Body->Comp5" bodies 24 removing the originals makes body 42 in component "Component''''"
copy_body "Body->Comp6" bodies 23 removing the originals makes body 43 in component "Component'''''"
copy_body "Body->Comp7" bodies 25 removing the originals makes body 44 in component "Component''''''"
copy_body "Body->Comp8" bodies 27 removing the originals makes body 45 in component "Component'''''''"
copy_body "Body->Comp9" bodies 28 removing the originals makes body 46 in component "Component''''''''"
copy_body "Body->Comp10" bodies 20 removing the originals makes body 47 in component "Component'''''''''"
copy_body "Body->Comp11" bodies 32 removing the originals makes body 48 in component "Component''''''''''"
copy_body "Body->Comp12" bodies 33 removing the originals makes body 49 in component "Component'''''''''''"
copy_body "Body->Comp13" bodies 34 removing the originals makes body 50 in component "Component''''''''''''"
copy_body "Body->Comp14" bodies 30 removing the originals makes body 51 in component "Component'''''''''''''"
copy_body "Body->Comp15" bodies 29 removing the originals makes body 52 in component "Component''''''''''''''"
copy_body "Body->Comp16" bodies 31 removing the originals makes body 53 in component "Component'''''''''''''''"
copy_body "Body->Comp17" bodies 3 removing the originals makes body 54 in component "Component''''''''''''''''"
copy_body "Body->Comp18" bodies 2 removing the originals makes body 55 in component "Component'''''''''''''''''"
copy_body "Body->Comp19" bodies 1 removing the originals makes body 56 in component "Component''''''''''''''''''"
copy_body "Body->Comp20" bodies 4 removing the originals makes body 57 in component "Component'''''''''''''''''''"
copy_body "Body->Comp21" bodies 5 removing the originals makes body 58 in component "Component''''''''''''''''''''"
copy_body "Body->Comp22" bodies 6 removing the originals makes body 59 in component "Component'''''''''''''''''''''"
copy_body "Body->Comp23" bodies 7 removing the originals makes body 60 in component "Component''''''''''''''''''''''"
copy_body "Body->Comp24" bodies 16 removing the originals makes body 61 in component "Component'''''''''''''''''''''''"
copy_body "Body->Comp25" bodies 13 removing the originals makes body 62 in component "Component''''''''''''''''''''''''"
copy_body "Body->Comp26" bodies 17 removing the originals makes body 63 in component "Component'''''''''''''''''''''''''"
copy_body "Body->Comp27" bodies 18 removing the originals makes body 64 in component "Component''''''''''''''''''''''''''"
copy_body "Body->Comp28" bodies 11 removing the originals makes body 65 in component "Component'''''''''''''''''''''''''''"
copy_body "Body->Comp29" bodies 14 removing the originals makes body 66 in component "Component''''''''''''''''''''''''''''"
copy_body "Body->Comp30" bodies 12 removing the originals makes body 67 in component "Component'''''''''''''''''''''''''''''"
copy_body "Body->Comp31" bodies 15 removing the originals makes body 68 in component "Component''''''''''''''''''''''''''''''"
copy_body "Body->Comp32" bodies 10 removing the originals makes body 69 in component "Component'''''''''''''''''''''''''''''''"
copy_body "Body->Comp33" bodies 8 removing the originals makes body 70 in component "Component''''''''''''''''''''''''''''''''"
copy_body "Body->Comp34" bodies 9 removing the originals makes body 71 in component "Component'''''''''''''''''''''''''''''''''"
copy_body "Body->Comp35" bodies 37 removing the originals makes body 72 in component "Component''''''''''''''''''''''''''''''''''"
copy_body "Body->Comp36" bodies 36 removing the originals makes body 73 in component "Component'''''''''''''''''''''''''''''''''''"
copy_body "Body->Comp37" bodies 35 removing the originals makes body 74 in component "Component''''''''''''''''''''''''''''''''''''"
sketch "Sketch16" plane through (0, 0, 0) normal (0, 1, 0) x (1, 0, 0)
  line L0 (-3269.792, -1354.9878) -> (-1899.2577, -1354.9878) construction
  line L1 (-1899.2577, -1354.9878) -> (-1899.2577, -2370.6516) construction
  line L2 (-1899.2577, -2370.6516) -> (-3269.792, -2370.6516) construction
  line L3 (-3269.792, -2370.6516) -> (-3269.792, -1354.9878) construction
  line L4 (-1899.2577, -2370.6516) -> (-1208.7394, -2370.6516)
  line L5 (-1208.7394, -2370.6516) -> (-1008.7907, -2121.4973)
  dimension "d221" = 76.2
  constraint coincident L1.end
  constraint perpendicular L1 L4
component "Component" placed x (1, 0, 0) y (0, 1, 0) z (0, 0, 1) at (0, 0, 0)
component "Component'" placed x (1, 0, 0) y (0, 1, 0) z (0, 0, 1) at (0, 0, 0)
component "Component''" placed x (1, 0, 0) y (0, 1, 0) z (0, 0, 1) at (0, 0, 0)
component "Component'''" placed x (1, 0, 0) y (0, 1, 0) z (0, 0, 1) at (0, 0, 0)
component "Component''''" placed x (1, 0, 0) y (0, 1, 0) z (0, 0, 1) at (0, 0, 0)
component "Component'''''" placed x (1, 0, 0) y (0, 1, 0) z (0, 0, 1) at (0, 0, 0)
component "Component''''''" placed x (1, 0, 0) y (0, 1, 0) z (0, 0, 1) at (0, 0, 0)
component "Component'''''''" placed x (1, 0, 0) y (0, 1, 0) z (0, 0, 1) at (0, 0, 0)
component "Component''''''''" placed x (1, 0, 0) y (0, 1, 0) z (0, 0, 1) at (0, 0, 0)
component "Component'''''''''" placed x (1, 0, 0) y (0, 1, 0) z (0, 0, 1) at (0, 0, 0)
component "Component''''''''''" placed x (1, 0, 0) y (0, 1, 0) z (0, 0, 1) at (0, 0, 0)
component "Component'''''''''''" placed x (1, 0, 0) y (0, 1, 0) z (0, 0, 1) at (0, 0, 0)
component "Component''''''''''''" placed x (1, 0, 0) y (0, 1, 0) z (0, 0, 1) at (0, 0, 0)